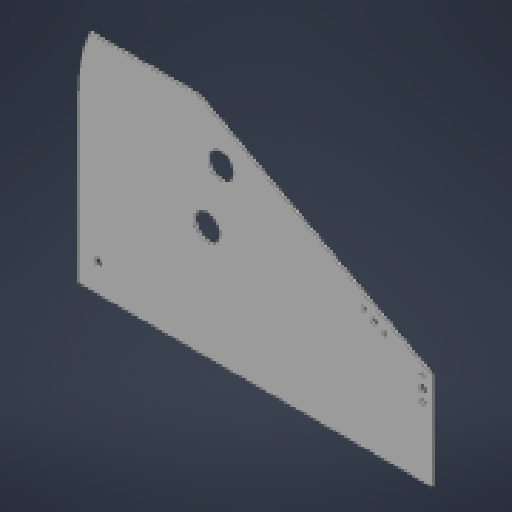
# Autodesk Inventor part: стенка
Saved by Autodesk Inventor 2025 (Build 290162000, 162)
## iProperties
Created: 2025-10-03
Part Number: стенка
Material: Типовые
Document SubType Name: Modeling
Designer: Phantom
Density: 1 g/cm^3
Appearance: По умолчанию
Author: Phantom
Autodesk Inventor part; units mm, degrees
ref_plane "YZ Plane" through (0, 0, 0) normal (1, 0, 0) x (0, 1, 0)
ref_plane "XZ Plane" through (0, 0, 0) normal (0, 1, 0) x (-1, 0, 0)
ref_plane "XY Plane" through (0, 0, 0) normal (0, 0, 1) x (1, 0, 0)
sketch "Эскиз1" plane through (0, 0, 0) normal (0, 0, 1) x (1, 0, 0)
  line L0 (0, 0) -> (380, 0)
  line L1 (380, 0) -> (380, 227)
  line L2 (380, 227) -> (0, 227)
  line L3 (0, 227) -> (0, 0)
  dimension "d0" = 380
  dimension "d1" = 227
  constraints: 8 end point, 2 parallel, 1 horizontal, 1 perpendicular
  measures "d0" distance of L2.end L1.end
  measures "d1" distance of L1.end L0.end
extrude "Выдавливание1" add sketch "Эскиз1" along normal blind 2
sketch "Эскиз2" plane through (0, 0, 2) normal (0, 0, 1) x (1, 0, 0)
  arc A0 (28.7106, 220.3235) -> (184.1593, 0) centre (184.1593, 165) ccw projected
  line L0 (380, 0) -> (380, 227) projected
  line L1 (380, 227) -> (0, 227) projected
  line L2 (0, 227) -> (0, 0) projected
  line L3 (0, 0) -> (380, 0) projected
  line L4 (19.1593, 227.9564) -> (19.1593, -26.9054)
  line L5 (0, 227) -> (0, 0) projected
  circle A1 centre (184.1593, 165) radius 165
  point P0 (19.1593, 165)
  point P1 (24, 227)
  point P2 (19.1593, 0)
  point P3 (19.1593, 227)
  point P4 (184.1593, 0)
  point P5 (28.7106, 220.3235)
  point P6 (31.2508, 227)
  constraints: 2 end point, 1 centre point, 1 coincident, 1 concentric, 1 parallel, 1 tangent
extrude "Выдавливание2" cut sketch "Эскиз2" against normal blind 10 contours A0 L4 L1 A1 | L4 L3 L2 L1
sketch "Эскиз3" plane through (0, 0, 0) normal (0, 0, -1) x (-1, 0, 0)
  line L0 (-232.105, -3.3128) -> (-396.3335, -92) projected
  line L1 (-142.3437, 227) -> (-503.0133, 32.2299)
  line L2 (-14.4537, 180) -> (-380, 180) projected
  line L3 (-14.4537, 180) -> (-380, 180) projected
  line L4 (-380, 0) -> (-380, 180) projected
  line L5 (-14.1593, 0) -> (-380, 0) projected
  line L6 (-14.1593, 0) -> (-14.1593, 170) projected
  arc A0 (-14.1593, 170) -> (-14.4537, 180) centre (-184.1593, 170) ccw projected
  line L7 (-19.1593, 0) -> (-19.1593, 165) projected
  arc A1 (-19.1593, 165) -> (-31.2508, 227) centre (-184.1593, 165) ccw projected
  line L8 (-380, 227) -> (-31.2508, 227) projected
  line L9 (-380, 0) -> (-380, 227) projected
  line L10 (-19.1593, 0) -> (-380, 0) projected
  point P0 (0, 0)
  point P1 (-380, 98.66)
  dimension "d6" = 160
  constraints: 2 end point, 1 parallel, 1 point on line, 1 other
  measures "d6" distance between parallel lines of L0 L1
extrude "Выдавливание3" cut sketch "Эскиз3" against normal blind 10 contours L1 L2 L9 L8 | L1 L4 L2
sketch "Эскиз4" plane through (0, 0, 0) normal (0, 0, -1) x (-1, 0, 0)
  circle A0 centre (-150.9975, 115.172) radius 3 projected
  circle A1 centre (-150.9975, 115.172) radius 3.1
  circle A2 centre (-184.1593, 165) radius 3.1 projected
  circle A3 centre (-184.1593, 165) radius 3.1
  arc A4 (-37.1443, 30.0275) -> (-37.7482, 26.6179) centre (-39.8587, 28.75) ccw projected
  circle A5 centre (-39.8587, 28.75) radius 3.5
  point P0 (0, 0)
  dimension "d9" = 6.2
  dimension "d10" = 6.2
  dimension "d11" = 7
  constraints: 3 centre point, 3 coincident
  measures "d9" diameter of A1
  measures "d10" diameter of A3
  measures "d11" diameter of A5
extrude "Выдавливание5" cut sketch "Эскиз4" against normal blind 10 contours A0 | A2 | A5
sketch "Эскиз5" plane through (0, 0, 0) normal (0, 0, -1) x (-1, 0, 0)
  circle A0 centre (-184.1593, 165) radius 3.1
  circle A1 centre (-185.6251, 167.2025) radius 3.5
  circle A2 centre (-150.9975, 115.172) radius 3 projected
  circle A3 centre (-150.9975, 115.172) radius 62.5
  circle A4 centre (-182.6583, 169.0593) radius 3.5
  line L0 (-182.6583, 169.0593) -> (-162.6583, 169.0593)
  line L1 (-182.6583, 169.0593) -> (-162.6583, 169.0593) construction
  line L2 (-162.6583, 169.0593) -> (-162.6583, 176.0593)
  line L3 (-162.6583, 176.0593) -> (-181, 176.0593)
  circle A5 centre (-165.1036, 176.0593) radius 3.5
  point P0 (0, 0)
  point P1 (-187.1037, 164.0302)
  point P2 (-182.1279, 167.3417)
  point P3 (-185.8413, 167.604)
  point P4 (-185.7497, 170.7003)
  dimension "d20" = 7
  dimension "d21" = 20
  dimension "d22" = 0
  dimension "d23" = 7
  dimension "d24" = 7
  constraints: 8 end point, 4 centre point, 3 point on circle, 2 horizontal, 2 perpendicular, 1 coincident, 1 collinear, 1 point on line, 6 other
  measures "d20" diameter of A4
  measures "d21" distance of L0.start L0.end
  measures "d22" distance between parallel lines of L0 L1
  measures "d23" distance of L0.end L2.end
  measures "d24" diameter of A5
extrude "Выдавливание6" cut sketch "Эскиз5" against normal blind 7 contours A4 A1 A0 | A0 A1 L0 A4 | A1 A3 A0 | A1 A4 A3 A0 | A0 A3 A1 | L0 A3 A4 | A3 A1 A4 A0 | A3 A4 A0 | A0 A4 A1 A3 | A1 A4 A3 | A5 L3 A3 | A3 L3 L2 A5 | L2 L3 A3 A5 | A3 L3 A5 picked at (-181.7788, 166.0755) picked at (-184.2655, 167.3284) picked at (-187.1066, 167.9908) picked at (-185.4271, 167.6129) picked at (-185.0911, 169.2148)
sketch "Эскиз6" plane through (0, 0, 0) normal (0, 0, -1) x (-1, 0, 0)
  circle A0 centre (-369.8544, 82.5008) radius 25
  circle A1 centre (-320.7436, 116.97) radius 25
  circle A2 centre (-369.8544, 82.5008) radius 3.1
  circle A3 centre (-320.7436, 116.97) radius 3.1
  point P0 (0, 0)
  dimension "d25" = 6.2
  dimension "d26" = 6.2
  constraints: 4 centre point, 2 coincident, 4 other
  measures "d25" diameter of A2
  measures "d26" diameter of A3
extrude "Выдавливание7" cut sketch "Эскиз6" against normal blind 7 contours A2 | A3
sketch "Эскиз7" plane through (0, 0, 0) normal (0, 0, -1) x (-1, 0, 0)
  arc A0 (-181.1878, 165.8832) -> (-185.7497, 170.7003) centre (-182.6583, 169.0593) ccw projected
  arc A1 (-187.1037, 164.0302) -> (-181.1878, 165.8832) centre (-184.1593, 165) ccw projected
  arc A2 (-185.7497, 170.7003) -> (-187.1037, 164.0302) centre (-185.6251, 167.2025) ccw projected
  point P0 (0, 0)
extrude "Выдавливание8" add sketch "Эскиз7" against normal up to surface (2 mm away)
sketch "Эскиз8" plane through (19.1593, 0, 0) normal (0, -1, 0) x (1, 0, 0)
  line L0 (0, 2) -> (0, 0) projected
  line L1 (0, 0) -> (360.8407, 0) projected
  line L2 (360.8407, 0) -> (360.8407, 2) projected
  line L3 (0, 2) -> (360.8407, 2) projected
  point P0 (-19.1593, 0)
extrude "Выдавливание9" cut sketch "Эскиз8" against normal blind 0.313
sketch "Эскиз9" plane through (0, 0, 0) normal (0, 0, -1) x (-1, 0, 0)
  circle A0 centre (-165.1036, 176.0593) radius 3.5 projected
  circle A1 centre (-165.1036, 176.0593) radius 12.6
  circle A2 centre (-150.9975, 115.172) radius 3 projected
  circle A3 centre (-150.9975, 115.172) radius 12.6
  line L0 (-320.7437, 116.97) -> (-310.185, 122.672)
  line L1 (-142.3437, 227) -> (-380, 98.66) projected
  line L2 (-320.7437, 116.97) -> (-331.3025, 111.268)
  line L3 (-380, 0.313) -> (-19.1593, 0.313) projected
  line L4 (-19.1593, 0.313) -> (-19.1593, 165) projected
  arc A4 (-19.1593, 165) -> (-31.2508, 227) centre (-184.1593, 165) ccw projected
  line L5 (-142.3437, 227) -> (-31.2508, 227) projected
  line L6 (-142.3437, 227) -> (-380, 98.66) projected
  line L7 (-380, 0.313) -> (-380, 98.66) projected
  circle A5 centre (-150.9975, 115.172) radius 3 projected
  circle A6 centre (-39.8587, 28.75) radius 3.5 projected
  circle A7 centre (-165.1036, 176.0593) radius 3.5 projected
  circle A8 centre (-369.8544, 82.5008) radius 3.1 projected
  circle A9 centre (-320.7436, 116.97) radius 3.1 projected
  circle A10 centre (-331.3025, 111.268) radius 2.1
  circle A11 centre (-310.185, 122.672) radius 2.1
  line L8 (-369.8544, 82.5008) -> (-369.8544, 94.5008)
  line L9 (-369.8544, 94.5008) -> (-369.8544, 70.5008)
  circle A12 centre (-369.8544, 94.5008) radius 2.1
  circle A13 centre (-369.8544, 70.5008) radius 2.1
  point P0 (0, 0)
  dimension "d33" = 25.2
  dimension "d34" = 25.2
  dimension "d35" = 12
  dimension "d36" = 12
  dimension "d37" = 4.2
  dimension "d38" = 4.2
  dimension "d39" = 12
  dimension "d40" = 24
  dimension "d41" = 4.2
  dimension "d42" = 4.2
  constraints: 8 end point, 6 centre point, 6 coincident, 1 collinear, 1 parallel, 1 point on line, 1 vertical, 1 other
  measures "d33" diameter of A1
  measures "d34" diameter of A3
  measures "d35" distance of L0.start L0.end
  measures "d36" distance of L0.start L2.end
  measures "d37" diameter of A10
  measures "d38" diameter of A11
  measures "d39" distance of L8.start L8.end
  measures "d40" distance of L8.end L9.end
  measures "d41" diameter of A12
  measures "d42" diameter of A13
extrude "Выдавливание10" cut sketch "Эскиз9" against normal through all contours A1 | A3 | A10 | A11 | A12 | A13
sketch "Эскиз10" plane through (0, 0, 0) normal (0, 0, -1) x (-1, 0, 0)
  line L0 (-0.0002, 0.3131) -> (-0.0002, 139.7466)
  arc A0 (-19.1593, 165) -> (-31.2508, 227) centre (-184.1593, 165) ccw projected
  line L1 (-19.1593, 0.313) -> (-19.1593, 165) projected
  line L2 (-0.0003, 0.313) -> (-0.0003, 165)
  arc A1 (-0.0003, 165) -> (-13.4958, 234.1991) centre (-184.1593, 165) ccw
  line L3 (-142.3437, 227) -> (-31.2508, 227) projected
  line L4 (-31.2508, 227) -> (23.6327, 227)
  line L5 (-19.1593, 0.313) -> (-0.0003, 0.313)
  point P0 (0, 0)
  point P1 (-10.7507, 227)
  dimension "d45" = 19.159
  constraints: 8 end point, 2 horizontal, 2 point on circle, 1 centre point, 1 vertical, 3 other
  measures "d45" distance between parallel lines of L1 L2
extrude "Выдавливание11" add sketch "Эскиз10" against normal up to surface (2 mm away)
sketch "Эскиз11" plane through (0, 0, 0) normal (0, 0, -1) x (-1, 0, 0)
  circle A0 centre (-310.185, 122.672) radius 2.1 projected
  circle A1 centre (-369.8544, 70.5008) radius 2.1 projected
  circle A2 centre (-165.1036, 176.0593) radius 12.6 projected
  circle A3 centre (-331.3025, 111.268) radius 2.1 projected
  circle A4 centre (-369.8544, 94.5008) radius 2.1 projected
  circle A5 centre (-150.9975, 115.172) radius 12.6 projected
  line L0 (-380, 0.313) -> (-0.0003, 0.313) projected
  line L1 (-0.0003, 0.313) -> (-0.0003, 165) projected
  arc A6 (-0.0003, 165) -> (-10.7507, 227) centre (-184.1593, 165) ccw projected
  line L2 (-10.7507, 227) -> (-142.3437, 227) projected
  line L3 (-142.3437, 227) -> (-380, 98.66) projected
  line L4 (-380, 0.313) -> (-380, 98.66) projected
  circle A7 centre (-39.8587, 28.75) radius 3.5 projected
  circle A8 centre (-369.8544, 82.5008) radius 3.1 projected
  circle A9 centre (-320.7436, 116.97) radius 3.1 projected
  arc A10 (-5.0003, 165) -> (-14.3095, 222) centre (-184.1593, 165) ccw
  line L5 (-5.0003, 165) -> (-5.0003, 5.313)
  line L6 (-5.0003, 5.313) -> (-375, 5.313)
  line L7 (-375, 5.313) -> (-375, 95.6776)
  line L8 (-375, 95.6776) -> (-141.0799, 222)
  line L9 (-141.0799, 222) -> (-14.3095, 222)
  line L10 (-150.9975, 115.172) -> (-150.9975, 5.313)
  line L11 (-165.1036, 176.0593) -> (-165.1036, 5.313)
  arc A11 (-334.838, 117.3661) -> (-313.3448, 128.9729) centre (-320.7436, 116.97) ccw
  arc A12 (-375, 69.3733) -> (-375, 95.6284) centre (-369.8544, 82.5008) ccw
  line L12 (-39.8587, 28.75) -> (-39.8587, 5.313)
  line L13 (-168.1036, 176.0593) -> (-168.1036, 5.313)
  line L14 (-162.1036, 176.0593) -> (-162.1036, 5.313)
  line L15 (-153.9975, 115.172) -> (-153.9975, 5.313)
  line L16 (-147.9975, 115.172) -> (-147.9975, 5.313)
  line L17 (-317.7436, 116.97) -> (-317.7436, 5.313)
  line L18 (-323.7436, 103.1928) -> (-323.7436, 5.313)
  line L19 (-366.8544, 82.5008) -> (-366.8544, 5.313)
  line L20 (-372.8544, 82.5008) -> (-372.8544, 5.313)
  line L21 (-36.8587, 28.75) -> (-36.8587, 5.313)
  line L22 (-42.8587, 28.75) -> (-42.8587, 5.313)
  line L23 (-369.8544, 82.5008) -> (-320.7436, 116.97)
  line L24 (-320.7436, 102.87) -> (-320.7436, 5.313)
  line L25 (-369.8544, 68.4008) -> (-369.8544, 5.313)
  line L26 (-368.131, 80.0453) -> (-319.0201, 114.5145)
  line L27 (-371.5779, 84.9564) -> (-322.467, 119.4255)
  line L28 (-150.9975, 115.172) -> (-320.7436, 116.97)
  line L29 (-165.1036, 176.0593) -> (-320.7436, 116.97)
  line L30 (-165.1036, 176.0593) -> (-150.9975, 115.172)
  line L31 (-150.9975, 115.172) -> (-39.8587, 28.75)
  line L32 (-165.1036, 176.0593) -> (-39.8587, 28.75)
  line L33 (-320.7436, 116.97) -> (-39.8587, 28.75)
  line L34 (-369.8544, 82.5008) -> (-39.8587, 28.75)
  point P0 (0, 0)
  dimension "d48" = 5
  dimension "d49" = 28.2
  dimension "d50" = 28.2
  dimension "d51" = 3
  dimension "d52" = 3
  dimension "d53" = 3
  dimension "d54" = 3
  dimension "d59" = 3
  dimension "d60" = 3
  dimension "d61" = 3
  dimension "d62" = 3
  constraints: 60 end point, 12 parallel, 10 point on line, 9 point on circle, 4 vertical, 3 centre point, 2 coincident, 1 perpendicular, 5 other
  measures "d48" radial gap between concentric circles of A6 A10
  measures "d49" diameter of A11
  measures "d50" diameter of A12
  measures "d51" distance between parallel lines of L11 L13
  measures "d52" distance between parallel lines of L11 L14
  measures "d53" distance between parallel lines of L10 L15
  measures "d54" distance between parallel lines of L10 L16
  measures "d59" distance between parallel lines of L12 L21
  measures "d60" distance between parallel lines of L12 L22
  measures "d61" distance between parallel lines of L23 L26
  measures "d62" distance between parallel lines of L23 L27
equation "\"d16\" = d24"
equation "\"d27\" = d24"
equation "\"d29\" = d24"
